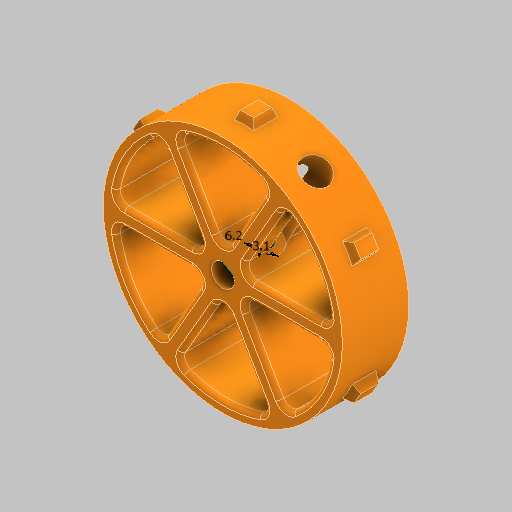
# Autodesk Inventor part: Self_wheel
Saved by Autodesk Inventor 2026 (Build 300175000, 175)
## iProperties
Created: 2026-06-08
Part Number: Self_wheel
Material: Типовые
Document SubType Name: Modeling
Designer: admin
Density: 1 g/cm^3
Appearance: Оранжевый
Author: admin
Autodesk Inventor part; units mm, degrees
ref_plane "YZ Plane" through (0, 0, 0) normal (1, 0, 0) x (0, 1, 0)
ref_plane "XZ Plane" through (0, 0, 0) normal (0, 1, 0) x (-1, 0, 0)
ref_plane "XY Plane" through (0, 0, 0) normal (0, 0, 1) x (1, 0, 0)
sketch "maun" plane through (0, 0, 0) normal (0, 0, 1) x (1, 0, 0)
  line L0 (12, 12) -> (-12, 12) construction
  line L1 (-12, 12) -> (-12, -12) construction
  line L2 (-12, -12) -> (12, -12) construction
  line L3 (12, -12) -> (12, 12) construction
  line L4 (12, 12) -> (-12, -12) construction
  line L5 (-12, 12) -> (12, -12) construction
  circle A0 centre (0, 0) radius 20
  circle A1 centre (0, 0) radius 31
  circle A2 centre (0, 0) radius 27
  dimension "d0" = 24
  dimension "d1" = 40
  dimension "d2" = 62
  dimension "d3" = 4
  constraints: 12 end point, 3 centre point, 3 coincident, 2 midpoint, 2 parallel, 2 perpendicular, 1 horizontal
  measures "d0" distance of L0.start L0.end
  measures "d1" diameter of A0
  measures "d2" diameter of A1
  measures "d3" radial gap between concentric circles of A1 A2
extrude "Выдавливание1" add sketch "maun" against normal blind 10 contours A0 | A2
extrude "Выдавливание2" add sketch "maun" along normal blind 5 contours A0 | A2
sketch "Эскиз7" plane through (0, 0, 5) normal (0, 0, 1) x (1, 0, 0)
  circle A0 centre (0, 0) radius 2.55
  line L0 (-0.2027, 2.5419) -> (2.3027, 1.0954)
  line L1 (0, 0) -> (2.55, 0) construction
  dimension "d98" = 5.1
  dimension "d99" = 0.45
  dimension "d100" = 30
  constraints: 4 end point, 3 point on circle, 1 centre point, 1 coincident, 1 horizontal
  measures "d98" diameter of A0
  measures "d99" distance edge to line of A0 L0
  measures "d100" angle of L1 L0
extrude "Выдавливание3" add sketch "maun" along normal up to surface (5 mm away) separate body contours A1
extrude "Выдавливание4" add sketch "maun" against normal up to surface (10 mm away) contours A1 bodies 2
ref_plane "РабПлоскость1" through (0, 0, -2.5) normal (0, 0, 1) x (1, 0, 0)
sketch "Эскиз2" plane through (0, 0, -2.5) normal (0, 0, 1) x (1, 0, 0)
  circle A0 centre (0, 0) radius 27 projected
  line L0 (2.1875, 26.9112) -> (1.5, 28.8)
  line L1 (1.5, 28.8) -> (0, 28.8)
  line L2 (0, 28.8) -> (0, 27) construction
  line L3 (-2.1875, 26.9112) -> (-1.5, 28.8)
  line L4 (-1.5, 28.8) -> (0, 28.8)
  arc A1 (2.1875, 26.9112) -> (-2.1875, 26.9112) centre (0, 0) ccw
  point P0 (-2.1875, 26.9112)
  dimension "d16" = 1.5
  dimension "d17" = 110
  dimension "d18" = 1.8
  constraints: 10 end point, 4 point on circle, 2 symmetric about line, 1 centre point, 1 coincident, 1 horizontal, 1 vertical, 1 vertical alignment
  measures "d16" distance of L0.end L1.end
  measures "d17" angle of L1 L0
  measures "d18" distance of L1.end L2.end
extrude "Выдавливание5" add sketch "Эскиз2" along normal mid plane 4 contours A0 L3 L4 L1 L0 bodies 1
draft "НаклГрань1" angle 20 pull direction (0, 1, 0) faces at (0.2433, 28.1967, -0.5) (0.2433, 28.1967, -4.5) fixed edges at (0, 28.8, -0.5) (0, 28.8, -4.5)
pattern_circular "Круговой массив1" count 6 over 360 about axis through (0, 0, 0) along (0, 0, -1) of "Выдавливание5", "НаклГрань1" bodies 1
fillet "Сопряжение1" radius 1.5 2 edges at (-31, 0, 5) (-31, 0, -10)
combine bodies "Комбинировать1" operation type subtract main body 2 bodies to subtract 1 keep tools yes
extrude "Выдавливание19" cut sketch "Эскиз7" against normal through all contours A0 L0 picked at (0.2036, 0.5225) bodies 1
sketch "Эскиз8" plane through (2.3027, 1.0954, -10) normal (-0.5, -0.8660254, 0) x (0.8660254, -0.5, 0)
  line L0 (0, 0) -> (-2.8931, 0) projected
  line L1 (0, 15) -> (0, 0) projected
  line L2 (-2.8931, 15) -> (0, 15) projected
  line L3 (-2.8931, 15) -> (-2.8931, 0) projected
  circle A0 centre (-1.4465, 7.5) radius 3.1
  circle A1 centre (-1.4465, 7.5) radius 1.55
  line L4 (-2.8931, 7.5) -> (0, 7.5) construction
  point P0 (-1.4465, 10)
  dimension "d103" = 3.1
  dimension "d104" = 6.2
  constraints: 3 midpoint, 2 centre point, 2 end point, 1 coincident
  measures "d103" diameter of A1
  measures "d104" diameter of A0
sketch "Эскиз9" plane through (0, 0, 5) normal (0, 0, 1) x (1, 0, 0)
  arc A0 (-0.2027, 2.5419) -> (2.3027, 1.0954) centre (0, 0) ccw projected
  circle A1 centre (0, 0) radius 27 projected
  circle A2 centre (0, 0) radius 5.05
  circle A3 centre (0, 0) radius 24.5
  line L0 (2.525, 4.3734) -> (12.25, 21.2176)
  line L1 (0, 0) -> (0, 24.5) construction
  line L2 (0.5865, 5.0158) -> (10.4771, 22.1468)
  line L3 (4.0506, 3.0158) -> (13.9412, 20.1468)
  line L4 (4.6371, 2) -> (24.4182, 2)
  dimension "d109" = 2.5
  dimension "d110" = 2.5
  dimension "d111" = 30
  dimension "d112" = 2
  dimension "d115" = 60
  constraints: 10 end point, 7 point on circle, 2 centre point, 2 coincident, 1 parallel, 1 point on line, 1 vertical, 5 other
  measures "d109" radial gap between concentric circles of A0 A2
  measures "d110" radial gap between concentric circles of A1 A3
  measures "d111" angle of L0 L1
  measures "d112" distance between parallel lines of L0 L2
extrude "Выдавливание22" cut sketch "Эскиз9" against normal through all contours A2 L3 A3 L4 bodies 1
fillet "Сопряжение8" radius 2 4 edges at (13.9412, 20.1468, -2.5) (24.4182, 2, -2.5) (4.0506, 3.0158, -2.5) (4.6371, 2, -2.5)
fillet "Сопряжение9" radius 1 12 edges at (14.1917, 19.1455, 5) (21.2176, 12.25, 5) (23.6764, 2.7176, 5) (14.534, 2, 5) (5.1953, 2.9995, 5) (8.9991, 11.5868, 5) (21.2176, 12.25, -10) (23.6764, 2.7176, -10) (14.534, 2, -10) (5.1953, 2.9995, -10) (8.9991, 11.5868, -10) (14.1917, 19.1455, -10)
pattern_circular "Круговой массив4" count 6 over 360 about axis through (0, 0, 0) along (0, 0, -1) of "Выдавливание22", "Сопряжение9", "Сопряжение8" bodies 1
extrude "Выдавливание23" cut sketch "Эскиз8" against normal through all contours A0 L3 A1 L1 | L1 A1 A0 | A0 L3 A1 | A1 L3 L1 | L1 A1 | A1 L3 | A0 L1 A1 L3 bodies 1
extrude "Выдавливание24" add sketch "Эскиз8" against normal up to surface (3.0421 mm away) contours A0 L3 A1 L1 | L1 A1 A0 | A0 L3 A1 | A0 L1 A1 L3 bodies 1
